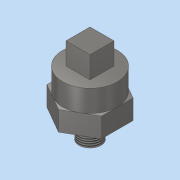
# Autodesk Inventor part: PressureSensor
Saved by Autodesk Inventor 2017 (Build 210142000, 142)
## iProperties
Created: 2018-02-06
Part Number: PressureSensor
Material: Steel, Carbon
Document SubType Name: Modeling
Designer: Derek Wider
Density: 1.93646 g/cm^3
Appearance: Semi-Polished
Mass: 22.6796 g
Surface Area: 34.8634 cm^2
Volume: 11.7119 cm^3
Author: Derek Wider
Autodesk Inventor part; units mm, degrees
ref_plane "XZ Plane" through (0, 0, 0) normal (0, 1, 0) x (-1, 0, 0)
ref_plane "XY Plane" through (0, 0, 0) normal (0, 0, 1) x (1, 0, 0)
sketch "Sketch2" plane through (0, 0, 0) normal (0, 1, 0) x (-1, 0, 0)
  circle A0 centre (0, 0) radius 5
  dimension "d0" = 10
  constraints: 1 centre point, 1 coincident
  measures "d0" diameter of A0
extrude "Extrusion1" add sketch "Sketch2" along normal blind 10
sketch "Sketch3" plane through (0, 10, 0) normal (0, 1, 0) x (1, 0, 0)
  line L0 (0, -14.4338) -> (-12.5, -7.2169)
  line L1 (-12.5, -7.2169) -> (-12.5, 7.2169)
  line L2 (-12.5, 7.2169) -> (0, 14.4338)
  line L3 (0, 14.4338) -> (12.5, 7.2169)
  line L4 (12.5, 7.2169) -> (12.5, -7.2169)
  line L5 (12.5, -7.2169) -> (0, -14.4338)
  point P0 (0, 0)
  point P1 (0, 0)
  dimension "d14" = 25
  constraints: 12 end point, 1 coincident, 13 other
  measures "d14" distance between parallel lines of L4 L1
extrude "Extrusion2" add sketch "Sketch3" along normal blind 9
sketch "Sketch4" plane through (0, 19, 0) normal (0, 1, 0) x (1, 0, 0)
  circle A0 centre (0, 0) radius 12.5
  line L0 (-12.5, -7.2169) -> (0, -14.4338) projected
  constraints: 1 centre point, 1 coincident, 1 tangent
extrude "Extrusion3" add sketch "Sketch4" along normal blind 10
sketch "Sketch5" plane through (0, 29, 0) normal (0, 1, 0) x (1, 0, 0)
  line L0 (5.5, -5.5) -> (-5.5, -5.5)
  line L1 (-5.5, -5.5) -> (-5.5, 5.5)
  line L2 (-5.5, 5.5) -> (5.5, 5.5)
  line L3 (5.5, 5.5) -> (5.5, -5.5)
  line L4 (5.5, -5.5) -> (-5.5, 5.5) construction
  line L5 (-5.5, -5.5) -> (5.5, 5.5) construction
  point P0 (0, 0)
  dimension "d7" = 11
  dimension "d8" = 11
  constraints: 12 end point, 2 midpoint, 2 parallel, 1 horizontal, 1 perpendicular
  measures "d7" distance of L1.end L2.end
  measures "d8" distance of L0.end L1.end
extrude "Extrusion4" add sketch "Sketch5" along normal blind 10
thread "Thread1" size "1/8" designation "1/8 - 27 NPT" standard "NPT for PVC Pipe and Fitting" length 9.967
sketch "Sketch8" plane through (0, 0, 0) normal (0, -1, 0) x (1, 0, 0)
  circle A0 centre (0, 0) radius 1.5
  dimension "d24" = 3
  constraints: 1 centre point, 1 coincident
  measures "d24" diameter of A0
extrude "Extrusion7" cut sketch "Sketch8" against normal blind 9
ref_plane "Work Plane1" through (0, 19, 0) normal (0.866, 0, 0.5) x (0, 1, 0)
equation "\"d8\" = d7"
body "Solid1"
